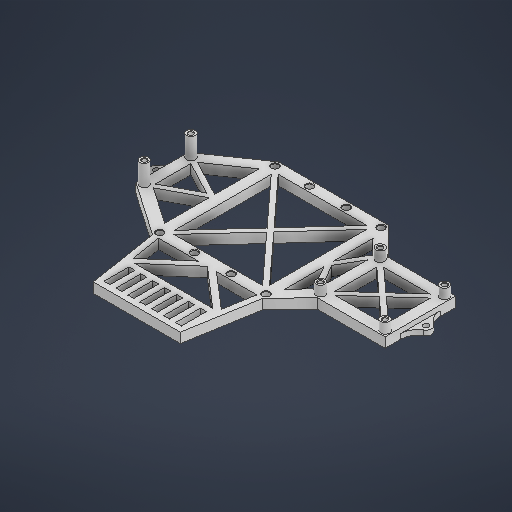
# Autodesk Inventor part: HolderForDriversNShit
Saved by Autodesk Inventor 2026.1 (Build 301233000, 233)
## iProperties
Created: 2026-06-25
Part Number: HolderForDriversNShit
Material: Generic
Document SubType Name: Modeling
Designer: Ru Racing
Density: 1 g/cm^3
Appearance: Default
Author: Ru Racing
Autodesk Inventor part; units mm, degrees
ref_plane "YZ Plane" through (0, 0, 0) normal (1, 0, 0) x (0, 1, 0)
ref_plane "XZ Plane" through (0, 0, 0) normal (0, 1, 0) x (-1, 0, 0)
ref_plane "XY Plane" through (0, 0, 0) normal (0, 0, 1) x (1, 0, 0)
sketch "TopViewPlanning Sketch" plane through (0, 0, 0) normal (0, 1, 0) x (-1, 0, 0)
  line L0 (53.5, -58) -> (18.5, -58) construction
  line L1 (18.5, -58) -> (18.5, 58) construction
  line L2 (18.5, 58) -> (53.5, 58) construction
  line L3 (53.5, 58) -> (53.5, -58) construction
  line L4 (-18.5, -58) -> (-53.5, -58) construction
  line L5 (-53.5, -58) -> (-53.5, 58) construction
  line L6 (-53.5, 58) -> (-18.5, 58) construction
  line L7 (-18.5, 58) -> (-18.5, -58) construction
  line L8 (18.5, 0) -> (-18.5, 0) construction
  line L9 (53.5, 0) -> (70.5, 0) construction
  line L10 (70.5, 0) -> (103.5, 0) construction
  line L11 (103.5, -23.5) -> (103.5, 23.5) construction
  line L12 (70.5, -51.5) -> (70.5, 51.5) construction
  line L13 (-53.5, 0) -> (-70.5, 0) construction
  line L14 (-70.5, -51.5) -> (-70.5, 51.5) construction
  line L15 (-70.5, 0) -> (-80.5, 0) construction
  line L16 (-80.5, 30) -> (-145.5, 30) construction
  line L17 (-145.5, 30) -> (-145.5, -30) construction
  line L18 (-145.5, -30) -> (-80.5, -30) construction
  line L19 (-80.5, -30) -> (-80.5, 30) construction
  point P0 (0, 0)
  point P1 (0, 0)
  dimension "Driver_WidthBetweenHoles" = 35
  dimension "Driver_WidthBetweenDrivers" = 37
  dimension "d4" = 17
  dimension "Driver_HeightBetweenHoles" = 116
  dimension "d6" = 33
  dimension "d7" = 103
  dimension "d8" = 47
  dimension "d10" = 10
  dimension "d30" = 65
  dimension "d31" = 60
  constraints: 40 end point, 15 coincident, 9 midpoint, 6 horizontal, 6 parallel, 3 equal length, 3 perpendicular, 3 point on line, 3 vertical
  measures "Driver_WidthBetweenHoles" distance of L0.start L0.end
  measures "Driver_WidthBetweenDrivers" distance of L8.start L8.end
  measures "d4" distance of L9.start L9.end
  measures "Driver_HeightBetweenHoles" distance of L4.end L5.end
  measures "d6" distance of L9.end L10.end
  measures "d7" distance of L12.start L12.end
  measures "d8" distance of L11.start L11.end
  measures "d10" distance of L15.end L13.end
  measures "d30" distance of L17.end L18.end
  measures "d31" distance of L16.end L17.end
sketch "Sketch2" plane through (0, 0, 0) normal (0, 1, 0) x (-1, 0, 0)
  circle A0 centre (103.5, -23.5) radius 5.5 construction
  circle A1 centre (53.5, -58) radius 5.5 construction
  circle A2 centre (18.5, -58) radius 5.5 construction
  circle A3 centre (-18.5, -58) radius 5.5 construction
  circle A4 centre (-53.5, -58) radius 5.5 construction
  line L0 (109, 0) -> (109, -26.3872)
  line L1 (109, -26.3872) -> (55.2134, -63.5)
  line L2 (55.2134, -63.5) -> (-55.837, -63.5)
  line L3 (51.7866, -52.5) -> (59, -47.5228) construction
  line L4 (98, -20.6128) -> (98, 0)
  line L5 (51.7866, -52.5) -> (48, -52.5) construction
  line L6 (78.5, -34.0678) -> (84.7472, -43.1217) construction
  line L7 (109, 0) -> (98, 0) construction
  circle A5 centre (-80.5, -30) radius 5.5 construction
  circle A6 centre (-145.5, -30) radius 5.5 construction
  line L8 (-55.837, -63.5) -> (-82.837, -35.5)
  line L9 (-82.837, -35.5) -> (-151, -35.5)
  line L10 (-78.163, -24.5) -> (-86, -24.5) construction
  line L11 (-51.163, -52.5) -> (-59, -44.3728) construction
  line L12 (-0.3118, -63.5) -> (-0.3118, -52.5) construction
  line L13 (-69.337, -49.5) -> (-61.4187, -41.8645) construction
  line L14 (-151, -35.5) -> (-151, 0)
  line L15 (-151, 0) -> (-140, 0) construction
  line L16 (-140, 0) -> (-140, -24.5)
  line L17 (98, 0) -> (-140, 0) construction
  line L18 (53.5, -58) -> (53.5, 0) construction
  line L19 (-53.5, -58) -> (-53.5, 0) construction
  line L20 (-80.5, -30) -> (-80.5, 0) construction
  line L21 (59, -47.5228) -> (59, 0)
  line L22 (48, -52.5) -> (48, -48.795) construction
  line L23 (-48, -52.5) -> (-48, -48.795) construction
  line L24 (-59, -44.3728) -> (-59, 0)
  line L25 (-75, -27.7802) -> (-75, 0)
  line L26 (-86, -24.5) -> (-86, 0)
  line L27 (59, -23.7614) -> (48, -23.7614) construction
  line L28 (-48, -24.3975) -> (-59, -24.3975) construction
  line L29 (-75, -13.8901) -> (-86, -13.8901) construction
  line L30 (48, -52.5) -> (44.6126, -52.5) construction
  line L31 (59, -47.5228) -> (98, -20.6128)
  line L32 (-48, -52.5) -> (-51.163, -52.5) construction
  line L33 (-59, -44.3728) -> (-75, -27.7802)
  line L34 (-75, -27.7802) -> (-78.163, -24.5) construction
  line L35 (-86, -24.5) -> (-140, -24.5)
  line L36 (109, 0) -> (109, 26.3872)
  line L37 (109, 26.3872) -> (55.2134, 63.5)
  line L38 (55.2134, 63.5) -> (-55.837, 63.5)
  line L39 (98, 20.6128) -> (98, 0)
  line L40 (-55.837, 63.5) -> (-82.837, 35.5)
  line L41 (-82.837, 35.5) -> (-151, 35.5)
  line L42 (-151, 35.5) -> (-151, 0)
  line L43 (-140, 0) -> (-140, 24.5)
  line L44 (59, 47.5228) -> (59, 0)
  line L45 (48, 52.5) -> (48, 48.795) construction
  line L46 (-48, 52.5) -> (-48, 48.795) construction
  line L47 (-59, 44.3728) -> (-59, 0)
  line L48 (-75, 27.7802) -> (-75, 0)
  line L49 (-86, 24.5) -> (-86, 0)
  line L50 (48, 52.5) -> (44.6126, 52.5) construction
  line L51 (59, 47.5228) -> (98, 20.6128)
  line L52 (-59, 44.3728) -> (-75, 27.7802)
  line L53 (-86, 24.5) -> (-140, 24.5)
  line L54 (48, -52.5) -> (-48, 52.5) construction
  line L55 (48, -48.795) -> (3.3874, 0)
  line L56 (44.6126, -52.5) -> (0, -3.705)
  line L57 (48, 48.795) -> (3.3874, 0)
  line L58 (-48, -48.795) -> (-3.3874, 0)
  line L59 (-48, -52.5) -> (48, 52.5) construction
  line L60 (0, -3.705) -> (-3.3874, 0) construction
  line L61 (-3.3874, 0) -> (-48, 48.795)
  line L62 (3.3874, 0) -> (0, 3.705) construction
  line L63 (0, 3.705) -> (-44.6126, 52.5)
  line L64 (-3.3874, 0) -> (0, 3.705) construction
  line L65 (0, 3.705) -> (44.6126, 52.5)
  line L66 (3.3874, 0) -> (0, -3.705) construction
  line L67 (0, -3.705) -> (-44.6126, -52.5)
  line L68 (22.3063, -28.1025) -> (25.9964, -24.7286) construction
  line L69 (44.6126, -52.5) -> (-44.6126, -52.5)
  line L70 (48, -48.795) -> (48, 0)
  line L71 (-44.6126, -52.5) -> (-48, -52.5) construction
  line L72 (-48, -48.795) -> (-48, 0)
  line L73 (-48, 48.795) -> (-48, 0)
  line L74 (-44.6126, 52.5) -> (-48, 52.5) construction
  line L75 (44.6126, 52.5) -> (-44.6126, 52.5)
  line L76 (48, 48.795) -> (48, 0)
  line L77 (98, -20.6128) -> (59, 0) construction
  line L78 (-75, -27.7802) -> (-59, 0) construction
  line L79 (-59, 0) -> (-75, 27.7802) construction
  line L80 (95.6794, -22.214) -> (59, -2.8277)
  line L81 (98, -17.7851) -> (64.3501, 0)
  line L82 (98, 17.7851) -> (64.3501, 0)
  line L83 (95.6794, 22.214) -> (59, 2.8277)
  line L84 (81.1751, -8.8925) -> (78.8386, -13.3131) construction
  line L85 (-73.1938, -29.6533) -> (-59, -5.0091)
  line L86 (-75, -22.7711) -> (-61.885, 0)
  line L87 (-61.885, 0) -> (-75, 22.7711)
  line L88 (-59, 5.0091) -> (-73.1938, 29.6533)
  line L89 (-68.4425, -11.3855) -> (-64.1098, -13.881) construction
  line L90 (98, 20.6128) -> (59, 0) construction
  line L91 (-86, -24.5) -> (-140, 24.5) construction
  line L92 (-140, -24.5) -> (-86, 24.5) construction
  line L93 (-86, -21.1242) -> (-109.2797, 0)
  line L94 (-109.2797, 0) -> (-86, 21.1242)
  line L95 (-89.7203, 24.5) -> (-113, 3.3758)
  line L96 (-113, 3.3758) -> (-136.2797, 24.5)
  line L97 (-140, 21.1242) -> (-116.7203, 0)
  line L98 (-140, -21.1242) -> (-116.7203, 0)
  line L99 (-136.2797, -24.5) -> (-113, -3.3758)
  line L100 (-113, -3.3758) -> (-89.7203, -24.5)
  line L101 (-97.6399, -10.5621) -> (-100.9998, -14.2649) construction
  point P0 (0, 0)
  point P1 (-53.5, 58)
  point P2 (-18.5, 58)
  point P3 (18.5, 58)
  point P4 (53.5, 58)
  point P5 (103.5, 23.5)
  point P6 (-145.5, 30)
  point P7 (-80.5, 30)
  dimension "d12" = 11
  dimension "d13" = 5
  dimension "d17" = 11
  constraints: 202 end point, 44 point on line, 32 parallel, 21 perpendicular, 14 vertical, 13 vertical alignment, 12 tangent, 10 equal length, 10 midpoint, 9 horizontal, 7 centre point, 7 coincident, 6 equal radius, 4 collinear, 31 other
  measures "d12" distance of L0.start L4.end
  measures "d13" distance of L68.start L68.end
  measures "d17" diameter of A0
extrude "Extrusion1" add sketch "Sketch2" against normal blind 10 contours L0 L1 L2 L8 L9 L14 L42 L41 L40 L38 L37 L36 | L31 L80 L21 L44 L83 L51 L39 L82 L81 L4 | L98 L97 L43 L53 L96 L95 L49 L94 L93 L26 L35 L100 L99 L16 | L85 L33 L25 L86 L87 L48 L52 L88 L47 L24
sketch "Sketch3" plane through (0, 0, 0) normal (0, 1, 0) x (1, 0, 0)
  circle A0 centre (-103.5, 23.5) radius 4.5
  circle A1 centre (-103.5, -23.5) radius 4.5
  point P0 (0, 0)
  dimension "d18" = 9
  constraints: 2 centre point, 2 coincident, 1 equal radius
  measures "d18" diameter of A0
extrude "Extrusion2" add sketch "Sketch3" along normal blind 21
sketch "Sketch4" plane through (-103.5, 21, -23.5) normal (0, 1, 0) x (1, 0, 0)
  point P0 (103.5, -23.5)
  point P1 (0, 0)
  point P2 (0, -47)
hole "Hole1" at (-103.5, 21, -23.5) at (-103.5, 21, 23.5) direction (0, -1, 0) diameter 4.6 depth 7 tip angle 120 countersink diameter 5.6 countersink angle 90
sketch "Sketch5" plane through (0, 0, 0) normal (0, 1, 0) x (1, 0, 0)
  point P0 (0, 0)
  point P1 (-53.5, 58)
  point P2 (53.5, 58)
  point P3 (18.5, 58)
  point P4 (-18.5, 58)
  point P5 (-53.5, -58)
  point P6 (-18.5, -58)
  point P7 (18.5, -58)
  point P8 (53.5, -58)
hole "Hole2" at (-53.5, 0, -58) at (53.5, 0, -58) at (18.5, 0, -58) at (-18.5, 0, -58) at (-53.5, 0, 58) at (-18.5, 0, 58) at (18.5, 0, 58) at (53.5, 0, 58) direction (0, -1, 0) diameter 6.8 depth 7 tip angle 120 countersink diameter 7.8 countersink angle 90
sketch "Sketch6" plane through (0, 0, 0) normal (0, 1, 0) x (1, 0, 0)
  circle A0 centre (80.5, 30) radius 4.5
  circle A1 centre (145.5, 30) radius 4.5
  circle A2 centre (145.5, -30) radius 4.5
  circle A3 centre (80.5, -30) radius 4.5
  point P0 (0, 0)
  dimension "d39" = 9
  constraints: 4 centre point, 4 coincident, 3 equal radius
  measures "d39" diameter of A0
extrude "Extrusion3" add sketch "Sketch6" along normal blind 10
sketch "Sketch7" plane through (80.5, 10, -30) normal (0, 1, 0) x (1, 0, 0)
  point P0 (-80.5, -30)
  point P1 (0, 0)
  point P2 (65, 0)
  point P3 (65, -60)
  point P4 (0, -60)
hole "Hole3" at (80.5, 10, -30) at (145.5, 10, -30) at (145.5, 10, 30) at (80.5, 10, 30) direction (0, -1, 0) diameter 4.6 depth 7 tip angle 120 countersink diameter 5.6 countersink angle 90
sketch "Sketch8" plane through (0, -10, 0) normal (0, -1, 0) x (1, 0, 0)
  line L0 (-55.2134, 63.5) -> (55.837, 63.5) projected
  line L1 (55.837, 63.5) -> (-55.2134, 63.5) projected
  line L2 (0, 103.5) -> (0, 128.5) construction
  line L3 (-3, 103.5) -> (-3, 128.5)
  line L4 (3, 103.5) -> (3, 128.5)
  line L5 (43.8407, 134.5) -> (-43.8407, 134.5)
  line L6 (0, 128.5) -> (0, 134.5) construction
  line L7 (0, 103.5) -> (0, 97.5) construction
  line L8 (49.7519, 63.5) -> (44.5915, 94.042)
  line L9 (44.0072, 97.5) -> (39.4143, 97.5) construction
  line L10 (-43.6908, 97.5) -> (-44.2479, 94.0221) construction
  line L11 (0, 97.5) -> (0, 63.5) construction
  line L12 (0, 59.538) -> (44.0072, 97.5) construction
  line L13 (0, 59.538) -> (-43.6908, 97.5) construction
  line L14 (44.5915, 94.042) -> (9.1858, 63.5)
  line L15 (-9.1197, 63.5) -> (-44.2479, 94.0221)
  line L16 (-39.1309, 97.5) -> (0, 63.5)
  line L17 (39.4143, 97.5) -> (0, 63.5)
  line L18 (19.7072, 80.5) -> (23.6263, 75.9568) construction
  line L19 (-3, 128.5) -> (3, 128.5)
  line L20 (-3, 103.5) -> (3, 103.5)
  line L21 (55.837, 63.5) -> (43.8407, 134.5)
  line L22 (-55.2134, 63.5) -> (-43.8407, 134.5)
  line L23 (43.8166, 193.8378) -> (183.959, -13.1891) construction
  line L24 (183.959, -13.1891) -> (-23.0678, -153.3315) construction
  line L25 (-23.0678, -153.3315) -> (-163.2102, 53.6954) construction
  line L26 (-163.2102, 53.6954) -> (43.8166, 193.8378) construction
  line L27 (43.8166, 193.8378) -> (-23.0678, -153.3315) construction
  line L28 (183.959, -13.1891) -> (-163.2102, 53.6954) construction
  line L29 (-43.6908, 97.5) -> (-49.6153, 98.449) construction
  line L30 (44.0072, 97.5) -> (49.9234, 98.4996) construction
  line L31 (-15, 103.5) -> (-15, 128.5)
  line L32 (-9, 103.5) -> (-9, 128.5)
  line L33 (9, 103.5) -> (9, 128.5)
  line L34 (15, 103.5) -> (15, 128.5)
  line L35 (-27, 103.5) -> (-27, 128.5)
  line L36 (-21, 103.5) -> (-21, 128.5)
  line L37 (21, 103.5) -> (21, 128.5)
  line L38 (27, 103.5) -> (27, 128.5)
  line L39 (-39, 103.5) -> (-39, 128.5)
  line L40 (-33, 103.5) -> (-33, 128.5)
  line L41 (33, 103.5) -> (33, 128.5)
  line L42 (39, 103.5) -> (39, 128.5)
  line L43 (-51, 103.5) -> (-51, 128.5)
  line L44 (-45, 103.5) -> (-45, 128.5)
  line L45 (45, 103.5) -> (45, 128.5)
  line L46 (51, 103.5) -> (51, 128.5)
  line L47 (-39, 103.5) -> (-33, 103.5)
  line L48 (-27, 103.5) -> (-21, 103.5)
  line L49 (-15, 103.5) -> (-9, 103.5)
  line L50 (-39, 128.5) -> (-33, 128.5)
  line L51 (-27, 128.5) -> (-21, 128.5)
  line L52 (-15, 128.5) -> (-9, 128.5)
  line L53 (9, 103.5) -> (15, 103.5)
  line L54 (15, 128.5) -> (9, 128.5)
  line L55 (27, 128.5) -> (21, 128.5)
  line L56 (21, 103.5) -> (27, 103.5)
  line L57 (33, 103.5) -> (39, 103.5)
  line L58 (39, 128.5) -> (33, 128.5)
  line L59 (-39.1309, 97.5) -> (-43.6908, 97.5) construction
  line L60 (39.4143, 97.5) -> (-39.1309, 97.5)
  line L61 (44.5915, 94.042) -> (44.0072, 97.5) construction
  line L62 (-44.2479, 94.0221) -> (-49.1369, 63.5)
  point P0 (0, 0)
  point P1 (-5, 63.5)
  point P2 (5, 63.5)
  point P3 (-9.1197, 63.5)
  point P4 (9.1858, 63.5)
  point P5 (10.3744, 20.2531)
  point P6 (151, -35.5)
  point P7 (151, 35.5)
  point P8 (-109, -26.3872)
  dimension "d63" = 40
  dimension "d65" = 6
  dimension "d66" = 25
  dimension "d67" = 250
  dimension "d71" = 12
  constraints: 122 end point, 17 point on line, 12 parallel, 11 perpendicular, 8 collinear, 8 equal length, 8 horizontal, 5 midpoint, 51 other
  measures "d63" distance from line of L2.start L0
  measures "d65" distance of L2.end L6.end
  measures "d66" distance of L3.start L3.end
  measures "d67" distance of L24.end L25.end
  measures "d71" distance of L3.start L31.start
extrude "Extrusion4" add sketch "Sketch8" against normal up to surface (10 mm away) contours L22 L5 L21 L0 L8 L14 L15 L62
sketch "Sketch10" plane through (0, -10, 0) normal (0, -1, 0) x (1, 0, 0)
  line L0 (-109, 26.3872) -> (-109, -26.3872) projected
  line L1 (151, -35.5) -> (151, 35.5) projected
  circle A0 centre (-114.75, 0) radius 2.75
  line L2 (-114.75, 0) -> (-112, 0) construction
  line L3 (-112, 0) -> (-109, 0) construction
  arc A1 (-117.625, -4.9796) -> (-117.625, 4.9796) centre (-114.75, 0) ccw construction
  arc A2 (-117.625, 4.9796) -> (-109, 19.9186) centre (-126.25, 19.9186) ccw
  arc A3 (-109, -19.9186) -> (-117.625, -4.9796) centre (-126.25, -19.9186) ccw
  line L4 (-117.625, -4.9796) -> (-109, -9.9593) construction
  arc A4 (-117.625, 4.9796) -> (-117.625, -4.9796) centre (-114.75, 0) ccw
  line L5 (21, 26.3872) -> (21, -26.3872) construction
  line L6 (-109, 0) -> (151, 0) construction
  circle A5 centre (156.75, 0) radius 2.75
  arc A6 (151, 19.9186) -> (159.625, 4.9796) centre (168.25, 19.9186) ccw
  arc A7 (159.625, -4.9796) -> (151, -19.9186) centre (168.25, -19.9186) ccw
  arc A8 (159.625, -4.9796) -> (159.625, 4.9796) centre (156.75, 0) ccw
  point P0 (0, 0)
  point P1 (21, 0)
  dimension "d76" = 5.5
  dimension "d77" = 3
  dimension "d78" = 60
  constraints: 14 point on circle, 10 end point, 8 centre point, 8 symmetric about line, 7 tangent, 4 midpoint, 3 point on line, 2 coincident, 1 collinear, 1 equal radius, 1 horizontal, 1 horizontal alignment, 1 parallel, 1 vertical, 6 other
  measures "d78" angle of L0 L4
extrude "Extrusion5" add sketch "Sketch10" against normal blind 5
equation "\"d12\" = d17"
equation "\"d39\" = d18"
equation "\"d42\" = d22"
equation "\"d46\" = d26"
equation "\"d48\" = d28"
equation "\"d44\" = d24"
equation "\"d47\" = d27"
equation "\"d22\" = 4.6"
equation "\"d26\" = 90deg"
equation "\"d28\" = 120deg"
equation "\"d24\" = 5.6"
equation "\"d27\" = 7"
body "Solid1"
